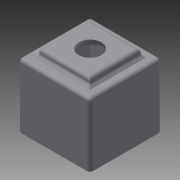
# Autodesk Inventor part: ceiling_mount
Saved by Autodesk Inventor 2014 (Build 180170000, 170)
## iProperties
Created: 2014-02-15
Part Number: ceiling_mount
Material: Generic
Document SubType Name: Modeling
Designer: anish
Density: 1 g/cm^3
Appearance: Default
Mass: 58.8955 g
Surface Area: 418.14 cm^2
Volume: 58.8955 cm^3
Author: anish
Autodesk Inventor part; units mm, degrees
ref_plane "YZ Plane" through (0, 0, 0) normal (1, 0, 0) x (0, 1, 0)
ref_plane "XZ Plane" through (0, 0, 0) normal (0, 1, 0) x (-1, 0, 0)
ref_plane "XY Plane" through (0, 0, 0) normal (0, 0, 1) x (1, 0, 0)
sketch "Sketch1" plane through (0, 0, 0) normal (0, 1, 0) x (-1, 0, 0)
  line L0 (0, 0) -> (68.58, 0)
  line L1 (68.58, 0) -> (68.58, 68.58)
  line L2 (68.58, 68.58) -> (0, 68.58)
  line L3 (0, 68.58) -> (0, 0)
  dimension "d2" = 68.58
  dimension "d3" = 68.58
  constraints: 8 end point, 2 parallel, 1 horizontal, 1 perpendicular
  measures "d2" distance between parallel lines of L1 L3
  measures "d3" distance between parallel lines of L0 L2
extrude "Extrusion1" add sketch "Sketch1" along normal blind 60.96
sketch "Sketch2" plane through (0, 0, 0) normal (0, -1, 0) x (1, 0, 0)
  line L0 (0, 0) -> (-68.58, 0) projected
  line L1 (0, 68.58) -> (0, 0) projected
  line L2 (-68.58, 68.58) -> (0, 68.58) projected
  line L3 (-68.58, 0) -> (-68.58, 68.58) projected
  line L4 (-66.04, 66.04) -> (-2.54, 66.04)
  line L5 (-2.54, 66.04) -> (-2.54, 2.54)
  line L6 (-2.54, 2.54) -> (-66.04, 2.54)
  line L7 (-66.04, 2.54) -> (-66.04, 66.04)
  dimension "d6" = 2.54
  dimension "d7" = 2.54
  dimension "d8" = 2.54
  dimension "d9" = 2.54
  constraints: 8 end point, 2 parallel, 1 horizontal, 1 perpendicular
  measures "d6" distance between parallel lines of L2 L4
  measures "d7" distance between parallel lines of L3 L7
  measures "d8" distance between parallel lines of L0 L6
  measures "d9" distance between parallel lines of L1 L5
extrude "Extrusion2" cut sketch "Sketch2" against normal blind 58.42 contours L4 L5 L6 L7
sketch "Sketch3" plane through (0, 60.96, 0) normal (0, 1, 0) x (1, 0, 0)
  line L0 (0, 0) -> (-68.58, 0) projected
  line L1 (-68.58, 0) -> (-68.58, -68.58) projected
  line L2 (-68.58, -68.58) -> (0, -68.58) projected
  line L3 (0, -68.58) -> (0, 0) projected
  line L4 (-58.42, -10.16) -> (-10.16, -10.16)
  line L5 (-10.16, -10.16) -> (-10.16, -58.42)
  line L6 (-10.16, -58.42) -> (-58.42, -58.42)
  line L7 (-58.42, -58.42) -> (-58.42, -10.16)
  dimension "d12" = 10.16
  dimension "d13" = 10.16
  dimension "d14" = 10.16
  dimension "d15" = 10.16
  constraints: 8 end point, 2 parallel, 1 horizontal, 1 perpendicular
  measures "d12" distance between parallel lines of L1 L7
  measures "d13" distance between parallel lines of L3 L5
  measures "d14" distance between parallel lines of L0 L4
  measures "d15" distance between parallel lines of L2 L6
extrude "Extrusion3" add sketch "Sketch3" along normal blind 7.366 contours L4 L5 L6 L7
sketch "Sketch4" plane through (0, 58.42, 0) normal (0, -1, 0) x (1, 0, 0)
  line L0 (-66.04, 2.54) -> (-66.04, 66.04) projected
  line L1 (-2.54, 2.54) -> (-66.04, 2.54) projected
  line L2 (-46.1963, 46.1962) -> (-22.3838, 46.1962)
  line L3 (-22.3838, 46.1962) -> (-22.3838, 22.3837)
  line L4 (-22.3838, 22.3837) -> (-46.1963, 22.3837)
  line L5 (-46.1963, 22.3837) -> (-46.1963, 46.1962)
  point P0 (0, 0)
  dimension "d18" = 23.8125
  dimension "d19" = 23.8125
  dimension "d20" = 19.8438
  dimension "d21" = 19.8438
  constraints: 8 end point, 2 parallel, 1 horizontal, 1 perpendicular
  measures "d18" distance between parallel lines of L3 L5
  measures "d19" distance of L2.end L3.end
  measures "d20" distance between parallel lines of L1 L4
  measures "d21" distance between parallel lines of L5 L0
extrude "Extrusion4" cut sketch "Sketch4" against normal blind 4.7625
sketch "Sketch5" plane through (0, 63.1825, 0) normal (0, -1, 0) x (1, 0, 0)
  line L0 (-46.1963, 46.1962) -> (-22.3838, 46.1962) projected
  line L1 (-22.3838, 22.3837) -> (-46.1963, 22.3837) projected
  line L2 (-22.3838, 46.1962) -> (-22.3838, 22.3837) projected
  arc A0 (-34.29, 22.3837) -> (-34.29, 46.1962) centre (-34.29, 34.29) ccw
  line L3 (-34.29, 46.1962) -> (-34.29, 22.3837)
  point P0 (0, 0)
  dimension "d24" = 23.8125
  dimension "d25" = 11.9062
  dimension "d26" = 23.8125
  constraints: 2 end point, 2 midpoint, 2 point on circle, 1 centre point
  measures "d24" diameter of A0
  measures "d25" distance from line of L2 A0.centre
  measures "d26" distance of L3.start L3.end
revolve "Revolution1" cut sketch "Sketch5" angle 360 about axis through (-34.29, 63.1825, 46.1962) along (0, 0, -1) contours A0 L3
sketch "Sketch6" plane through (-68.58, 0, 0) normal (-1, 0, 0) x (0, 0, 1)
  line L0 (0, 0) -> (68.58, 0) projected
  line L1 (68.58, 0) -> (68.58, 60.96) projected
  line L2 (0, 0) -> (0, 60.96) projected
  line L3 (68.58, 5.08) -> (60.96, 5.08)
  line L4 (60.96, 5.08) -> (60.96, 2.54)
  line L5 (60.96, 2.54) -> (68.58, 2.54)
  line L6 (68.58, 2.54) -> (68.58, 5.08)
  line L7 (68.58, 7.62) -> (0, 7.62)
  line L8 (0, 5.08) -> (7.62, 5.08)
  line L9 (7.62, 5.08) -> (7.62, 2.54)
  line L10 (7.62, 2.54) -> (0, 2.54)
  line L11 (0, 2.54) -> (0, 5.08)
  line L12 (2.54, 7.62) -> (2.54, 5.08)
  line L13 (2.54, 2.54) -> (2.54, 0)
  line L14 (66.04, 5.08) -> (66.04, 7.62)
  line L15 (66.04, 2.54) -> (66.04, 0)
  dimension "d28" = 2.54
  dimension "d29" = 2.54
  dimension "d30" = 2.54
  dimension "d31" = 7.62
  dimension "d32" = 2.54
  dimension "d33" = 2.54
  dimension "d34" = 7.62
  dimension "d35" = 2.54
  dimension "d36" = 2.54
  dimension "d37" = 2.54
  dimension "d38" = 2.54
  constraints: 26 end point, 12 point on line, 7 perpendicular, 4 parallel, 2 horizontal
  measures "d28" distance between parallel lines of L0 L5
  measures "d29" distance of L3.end L4.end
  measures "d30" distance between parallel lines of L3 L7
  measures "d31" distance between parallel lines of L1 L4
  measures "d32" distance between parallel lines of L0 L10
  measures "d33" distance between parallel lines of L7 L8
  measures "d34" distance between parallel lines of L11 L9
  measures "d35" distance between parallel lines of L12 L2
  measures "d36" distance between parallel lines of L2 L13
  measures "d37" distance between parallel lines of L1 L14
  measures "d38" distance between parallel lines of L1 L15
extrude "Extrusion5" cut sketch "Sketch6" against normal blind 66.04 contours L13 L10 L9 L8 L12 L7 L14 L3 L4 L5 L15 L0
sketch "Sketch7" plane through (-66.04, 2.54, 66.04) normal (1, 0, 0) x (0, 0, -1)
  line L0 (0, 2.54) -> (5.08, 2.54)
  line L1 (5.08, 2.54) -> (5.08, 0)
  line L2 (5.08, 0) -> (0, 0)
  line L3 (0, 0) -> (0, 2.54)
  point P0 (66.04, -2.54)
  constraints: 8 end point, 2 parallel, 1 horizontal, 1 perpendicular
extrude "Extrusion6" add sketch "Sketch7" along normal blind 66.04
sketch "Sketch8" plane through (-66.04, 2.54, 7.62) normal (1, 0, 0) x (0, 0, -1)
  line L0 (0, 2.54) -> (5.08, 2.54)
  line L1 (5.08, 2.54) -> (5.08, 0)
  line L2 (5.08, 0) -> (0, 0)
  line L3 (0, 0) -> (0, 2.54)
  point P0 (7.62, -2.54)
  constraints: 8 end point, 2 parallel, 1 horizontal, 1 perpendicular
extrude "Extrusion7" add sketch "Sketch8" along normal blind 66.04
chamfer "Chamfer1" distance 2.54 angle 45 4 edges at (-34.29, 60.96, 58.42) (-58.42, 60.96, 34.29) (-34.29, 60.96, 10.16) (-10.16, 60.96, 34.29)
fillet "Fillet1" radius 3.175 4 edges at (-10.16, 63.5, 34.29) (-34.29, 63.5, 58.42) (-58.42, 63.5, 34.29) (-34.29, 63.5, 10.16)
sketch "Sketch9" plane through (0, 58.42, 0) normal (0, -1, 0) x (1, 0, 0)
  line L0 (-46.1963, 22.3837) -> (-46.1963, 46.1962) projected
  line L1 (-46.1963, 46.1962) -> (-22.3838, 46.1962) projected
  line L2 (-22.3838, 46.1962) -> (-22.3838, 22.3837) projected
  line L3 (-22.3838, 22.3837) -> (-46.1963, 22.3837) projected
  line L4 (-66.04, 66.04) -> (-2.54, 66.04) projected
  line L5 (-66.04, 2.54) -> (-66.04, 66.04) projected
  line L6 (-2.54, 2.54) -> (-66.04, 2.54) projected
  line L7 (-2.54, 66.04) -> (-2.54, 2.54) projected
  line L8 (-53.34, 53.34) -> (-15.24, 53.34)
  line L9 (-15.24, 53.34) -> (-15.24, 15.24)
  line L10 (-15.24, 15.24) -> (-53.34, 15.24)
  line L11 (-53.34, 15.24) -> (-53.34, 53.34)
  point P0 (0, 0)
  dimension "d49" = 12.7
  dimension "d51" = 12.7
  dimension "d52" = 12.7
  dimension "d53" = 12.7
  constraints: 8 end point, 2 parallel, 1 horizontal, 1 perpendicular
  measures "d49" distance between parallel lines of L11 L5
  measures "d51" distance between parallel lines of L7 L9
  measures "d52" distance between parallel lines of L8 L4
  measures "d53" distance between parallel lines of L10 L6
extrude "Extrusion8" cut sketch "Sketch9" against normal blind 4.7625 contours L8 L9 L10 L11
fillet "Fillet2" radius 3.175 12 edges at (-68.58, 30.48, 0) (-68.58, 60.96, 34.29) (-34.29, 60.96, 0) (0, 30.48, 0) (0, 60.96, 34.29) (0, 30.48, 68.58) (-34.29, 60.96, 68.58) (-68.58, 30.48, 68.58) (-34.29, 68.326, 10.16) (-58.42, 68.326, 34.29) (-34.29, 68.326, 58.42) (-10.16, 68.326, 34.29)
body "Solid1"
